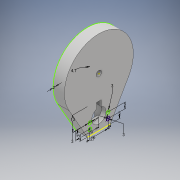
# Autodesk Inventor part: BasePart
Saved by Autodesk Inventor 2018 (Build 220112000, 112)
## iProperties
Created: 2019-10-08
Part Number: BasePart
Material: 一般
Document SubType Name: Modeling
Designer: Eiji Nishizawa
Density: 1 g/cm^3
Appearance: 既定
Mass: 23.0401 g
Surface Area: 97.2551 cm^2
Volume: 23.0401 cm^3
Author: Eiji Nishizawa
Autodesk Inventor part; units mm, degrees
note: some values were not read from the file. Chosen so that the rebuilt part matches the saved one: sketch regions of "押し出し8".
ref_plane "YZ Plane" through (0, 0, 0) normal (1, 0, 0) x (0, 1, 0)
ref_plane "XZ Plane" through (0, 0, 0) normal (0, 1, 0) x (-1, 0, 0)
ref_plane "XY Plane" through (0, 0, 0) normal (0, 0, 1) x (1, 0, 0)
sketch "スケッチ1" plane through (0, 0, 0) normal (1, 0, 0) x (0, 1, 0)
  circle A0 centre (0, 0) radius 30
  line L0 (10, -28.2843) -> (10, -43)
  line L1 (10, -43) -> (-10, -43)
  line L2 (-10, -43) -> (-10, -28.2843)
  line L3 (10, -43) -> (25.9808, -15)
  line L4 (-10, -43) -> (-25.9808, -15)
  circle A1 centre (0, 0) radius 2.35
  circle A2 centre (0, 0) radius 28
  point P0 (0, -30)
  point P1 (0, -28.05)
  point P2 (0, -26.4333)
  dimension "d2" = 20
  dimension "d10" = 4.7
  dimension "d34" = 13
  dimension "d39" = 2
  constraints: 10 end point, 5 point on circle, 3 centre point, 3 coincident, 1 parallel
  measures "d2" distance of L0.end L1.end
  measures "d10" diameter of A1
  measures "d34" distance edge to line of A0 L1
  measures "d39" radial gap between concentric circles of A0 A2
extrude "押し出し8" add sketch "スケッチ1" along normal blind 10 contours A0 | A0 L2 L4 | L3 L0 A0 | A0 L0 L1 L2 | A2
extrude "押し出し9" cut sketch "スケッチ1" along normal blind 3 contours A2
sketch "スケッチ3" plane through (0, 0, 0) normal (-1, 0, 0) x (0, 0, 1)
  line L0 (-15.35, 6.25) -> (-38, 6.25)
  line L1 (-38, 6.25) -> (-38, -6.25)
  line L2 (-38, -6.25) -> (-15.35, -6.25)
  line L3 (-15.35, -6.25) -> (-15.35, 6.25)
  line L4 (-15.35, 6.25) -> (-38, -6.25) construction
  line L5 (-38, 6.25) -> (-15.35, -6.25) construction
  line L6 (-15.35, -6.25) -> (-10.35, -6.25)
  line L7 (-10.35, -6.25) -> (-10.35, 6.25)
  line L8 (-10.35, 6.25) -> (-15.35, 6.25)
  line L9 (-15.35, 6.25) -> (-15.35, -6.25)
  line L10 (-38, -6.25) -> (-43, -6.25)
  line L11 (-43, -6.25) -> (-43, 6.25)
  line L12 (-43, 6.25) -> (-38, 6.25)
  line L13 (-38, 6.25) -> (-38, -6.25)
  circle A0 centre (-31.75, 0) radius 6.25
  circle A1 centre (-31.75, 0) radius 2.4
  line L14 (-43, -10) -> (-43, 10) projected
  point P0 (0, 0)
  point P1 (-26.675, 0)
  dimension "d42" = 22.65
  dimension "d43" = 12.5
  dimension "d44" = 5
  dimension "d45" = 5
  dimension "d46" = 12.5
  dimension "d47" = 0
  dimension "d48" = 4.8
  dimension "d49" = 0
  dimension "d50" = 0
  constraints: 28 end point, 6 parallel, 3 horizontal, 3 perpendicular, 2 centre point, 2 midpoint, 2 point on line, 1 coincident, 1 tangent
  measures "d42" distance between parallel lines of L3 L1
  measures "d43" distance of L2.end L0.start
  measures "d44" distance of L2.end L6.end
  measures "d45" distance of L1.end L10.end
  measures "d46" diameter of A0
  measures "d47" distance edge to line of A0 L1
  measures "d48" diameter of A1
  measures "d49" distance between parallel lines of L14 L11
  measures "d50" vertical distance of point (0, 0) A0.centre
extrude "押し出し10" cut sketch "スケッチ3" against normal blind 10 contours A0
extrude "押し出し11" cut sketch "スケッチ3" against normal blind 10 contours A1
extrude "押し出し12" cut sketch "スケッチ3" against normal blind 6 contours L3 L2 A0 L0 | A0 L1 L0 | A0 L2 L1
extrude "押し出し13" cut sketch "スケッチ3" against normal blind 3 contours L1 L10 L11 L12
sketch "スケッチ5" plane through (10, 0, 0) normal (1, 0, 0) x (0, 0, -1)
  arc A0 (31.75, 6.25) -> (31.75, -6.25) centre (31.75, 0) ccw projected
  line L0 (25.8286, -2) -> (20.8286, -2)
  line L1 (20.8286, -2) -> (20.8286, 2)
  line L2 (20.8286, 2) -> (25.8286, 2)
  line L3 (25.8286, 2) -> (25.8286, -2)
  point P0 (0, 0)
  dimension "d63" = 4
  dimension "d64" = 2
  dimension "d65" = 5
  constraints: 8 end point, 2 parallel, 1 horizontal, 1 perpendicular, 1 point on circle
  measures "d63" distance of L0.end L1.end
  measures "d64" distance from line of point (0, 0) L2
  measures "d65" distance of L1.end L2.end
extrude "押し出し14" cut sketch "スケッチ5" against normal blind 10
sketch "スケッチ6" plane through (10, 0, 0) normal (1, 0, 0) x (0, 0, -1)
  circle A0 centre (38, -8) radius 1.5
  circle A1 centre (38, 8) radius 1.5
  line L0 (43, -10) -> (43, 10) projected
  circle A2 centre (33, -8) radius 1.5
  circle A3 centre (33, 8) radius 1.5
  point P0 (0, 0)
  dimension "d68" = 5
  dimension "d69" = 5
  dimension "d74" = 3
  dimension "d76" = 16
  dimension "d77" = 2
  dimension "d78" = 2
  dimension "d81" = 3
  dimension "d82" = 5
  dimension "d83" = 5
  dimension "d84" = 3
  constraints: 4 centre point
  measures "d68" distance from line of A0.centre L0
  measures "d69" distance from line of L0 A1.centre
  measures "d74" diameter of A1
  measures "d76" distance of A0.centre A1.centre
  measures "d77" vertical distance of L0.end A1.centre
  measures "d78" vertical distance of L0.start A0.centre
  measures "d81" diameter of A3
  measures "d82" distance of A1.centre A3.centre
  measures "d83" distance of A0.centre A2.centre
  measures "d84" diameter of A2
extrude "押し出し15" cut sketch "スケッチ6" against normal blind 100 contours A0 | A1
extrude "押し出し16" cut sketch "スケッチ6" against normal blind 100 contours A2 | A3
